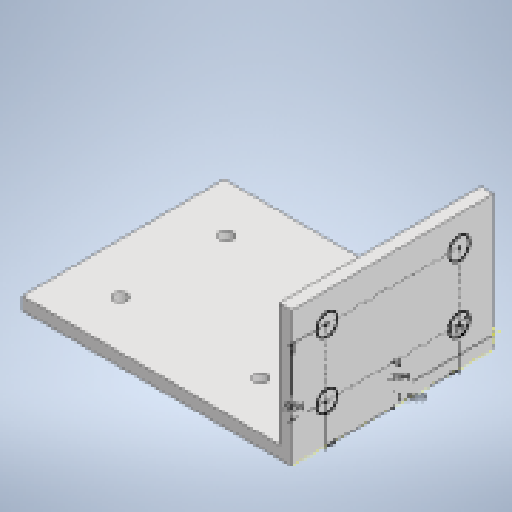
# Autodesk Inventor part: L_Bracketr
Saved by Autodesk Inventor 2023 (Build 270158000, 158)
## iProperties
Created: 2022-05-04
Part Number: L_Bracketr
Material: Generic
Document SubType Name: Modeling
Designer: plebbb
Density: 1 g/cm^3
Appearance: Default
Author: plebbb
Autodesk Inventor part; units mm, degrees
ref_plane "YZ Plane" through (0, 0, 0) normal (1, 0, 0) x (0, 1, 0)
ref_plane "XZ Plane" through (0, 0, 0) normal (0, 1, 0) x (-1, 0, 0)
ref_plane "XY Plane" through (0, 0, 0) normal (0, 0, 1) x (1, 0, 0)
sketch "Sketch1" plane through (0, 0, 0) normal (0, 0, 1) x (1, 0, 0)
  line L0 (0, 0) -> (101.6, 0)
  line L1 (101.6, 0) -> (101.6, 50.8)
  line L2 (0, 0) -> (0, 4.7625)
  line L3 (0, 4.7625) -> (96.8375, 4.7625)
  line L4 (96.8375, 4.7625) -> (96.8375, 50.8)
  line L5 (96.8375, 50.8) -> (101.6, 50.8)
  dimension "d0" = 101.6
  dimension "d1" = 50.8
  dimension "d2" = 4.7625
  constraints: 12 end point, 5 perpendicular, 1 horizontal, 1 vertical
  measures "d0" distance of L0.start L0.end
  measures "d1" distance of L0.end L1.end
  measures "d2" distance of L0.start L2.end
extrude "Extrusion1" add sketch "Sketch1" along normal blind 76.2
sketch "Sketch2" plane through (0, 0, 0) normal (0, -1, 0) x (1, 0, 0)
  line L0 (18.9, 18.1) -> (71.9, 18.1) construction
  line L1 (71.9, 18.1) -> (71.9, 58.1) construction
  line L2 (71.9, 58.1) -> (18.9, 58.1) construction
  line L3 (18.9, 58.1) -> (18.9, 18.1) construction
  line L4 (101.6, 0) -> (101.6, 76.2) construction
  circle A0 centre (18.9, 58.1) radius 2.5
  circle A1 centre (18.9, 18.1) radius 2.5
  circle A2 centre (71.9, 58.1) radius 2.5
  circle A3 centre (71.9, 18.1) radius 2.5
  point P0 (0, 0)
  point P1 (45.4, 58.1)
  point P2 (71.9, 38.1)
  point P3 (101.6, 38.1)
  dimension "d5" = 53
  dimension "d6" = 40
  dimension "d7" = 56.2
  dimension "d8" = 5
  constraints: 8 end point, 4 centre point, 3 coincident, 3 equal radius, 3 midpoint, 2 parallel, 1 horizontal, 1 horizontal alignment, 1 perpendicular
  measures "d5" distance of L1.end L2.end
  measures "d6" distance of L0.end L1.end
  measures "d7" horizontal distance of L4.end point (45.4, 58.1)
  measures "d8" diameter of A0
extrude "Extrusion2" cut sketch "Sketch2" against normal up to surface (4.7625 mm away)
sketch "Sketch3" plane through (101.6, 0, 0) normal (1, 0, 0) x (0, 0, -1)
  line L0 (-15.1, 14.7625) -> (-61.1, 14.7625) construction
  line L1 (-61.1, 14.7625) -> (-61.1, 39.7625) construction
  line L2 (-61.1, 39.7625) -> (-15.1, 39.7625) construction
  line L3 (-15.1, 39.7625) -> (-15.1, 14.7625) construction
  line L4 (0, 0) -> (-76.2, 0) construction
  circle A0 centre (-15.1, 14.7625) radius 4
  circle A1 centre (-15.1, 39.7625) radius 4
  circle A2 centre (-61.1, 14.7625) radius 4
  circle A3 centre (-61.1, 39.7625) radius 4
  point P0 (0, 4.7625)
  point P1 (-38.1, 14.7625)
  point P2 (-38.1, 0)
  dimension "d11" = 46
  dimension "d12" = 25
  dimension "d13" = 10
  dimension "d14" = 8
  constraints: 8 end point, 4 centre point, 4 coincident, 3 equal radius, 2 midpoint, 2 parallel, 1 horizontal, 1 perpendicular, 1 vertical alignment
  measures "d11" distance of L0.start L0.end
  measures "d12" distance of L0.end L1.end
  measures "d13" distance from line of L0 point (0, 4.763)
  measures "d14" diameter of A0
extrude "Extrusion3" cut sketch "Sketch3" against normal blind 25.4
body "Solid1"
